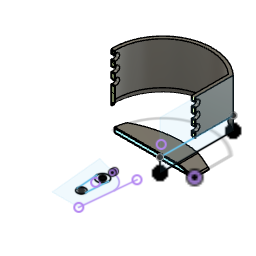
not a trashcan too v102 (Autodesk Fusion 360 design; units mm, degrees)
Autodesk Fusion 360 part; units mm, degrees
sketch "Sketch1" plane through (0, 0, 0) normal (0, 1, 0) x (1, 0, 0)
  circle A0 centre (0, 0) radius 35
  circle A1 centre (0, 0) radius 37.5
  line L0 (23, -29.6184) -> (23, 29.6184)
  line L1 (25.5, 27.4955) -> (25.5, -27.4955)
  dimension "d1" = 70
  dimension "d2" = 75
  dimension "d148" = 2.5
  dimension "d149" = 23
  constraint coincident A0.centre A1.centre
  constraint coincident A1 L0.start
  constraint coincident A1 L0.end
  constraint vertical L0
  constraint coincident A1 L1.start
  constraint coincident A1 L1.end
  constraint parallel L0 L1
  measures "d1" diameter of A0
  measures "d2" diameter of A1
  measures "d148" distance of L0 L1
  measures "d149" distance of A0.centre L0
extrude "Extrude1" add sketch "Sketch1" along normal blind 50 contours A0 L0 L1 | A0 A1 L0 L1 | A0 A1 L0 L1 | A0 A1 L0 makes body 1
ref_plane "WorkPlane2" through (0, 14, 0) normal (0, 1, 0) x (0, 0, 1)
sketch "Sketch4" plane through (0, 14, 0) normal (0, 1, 0) x (1, 0, 0)
  circle A0 centre (0, -68.5) radius 1.15
  circle A1 centre (0, -40.5) radius 1.15
  line L0 (-10, -36.1421) -> (10, -36.1421)
  line L1 (-10, -36.1421) -> (-10, -76.1421)
  line L2 (-10, -76.1421) -> (10, -76.1421)
  line L3 (10, -76.1421) -> (10, -36.1421)
  line L4 (-6.5, -43) -> (6.5, -43)
  line L5 (6.5, -43) -> (6.5, -66)
  line L6 (6.5, -66) -> (-6.5, -66)
  line L7 (-6.5, -66) -> (-6.5, -43)
  arc A2 (25.5, 27.4955) -> (25.5, -27.4955) centre (0, 0) ccw
  arc A3 (23, 26.3818) -> (23, -26.3818) centre (0, 0) ccw
  dimension "d28" = 2.3
  dimension "d29" = 2.3
  dimension "d30" = 28
  dimension "d33" = 40.5
  dimension "d36" = 20
  dimension "d37" = 40
  dimension "d38" = 10
  dimension "d39" = 10
  dimension "d40" = 13
  dimension "d41" = 23
  dimension "d42" = 3.5
  dimension "d43" = 2.5
  constraint coincident L0.start A2
  constraint coincident L0.end A2
  constraint horizontal L0
  constraint perpendicular L0 L1
  constraint perpendicular L1 L2
  constraint perpendicular L0 L3
  constraint horizontal L4
  constraint vertical L5
  constraint perpendicular L5 L6
  constraint perpendicular L4 L7
  measures "d28" diameter of A0
  measures "d29" diameter of A1
  measures "d30" distance of A0.centre A1.centre
  measures "d33" vertical distance of A1.centre A2.centre
  measures "d36" distance of L0.start L0.end
  measures "d37" distance of L0.start L1.end
  measures "d38" horizontal distance of A1.centre L0.start
  measures "d39" horizontal distance of A0.centre L0.start
  measures "d40" distance of L4.start L4.end
  measures "d41" distance of L4.end L5.end
  measures "d42" distance of L1 L7
  measures "d43" distance of A1.centre L4
extrude "Extrude2" add sketch "Sketch4" along normal blind 4 contours L1 L2 L3 A2 bodies 1
other "Base Mesh Feature1"
copy_body "Body->Comp1" bodies 1 removing the originals makes body 2 in component "Component"
ref_plane "WorkPlane3" through (0, -0.1, 0) normal (0, 1, 0) x (0, 0, 1)
sketch "Sketch8" plane through (0, -0.1, 0) normal (0, 1, 0) x (1, 0, 0)
  circle A0 centre (0, 0) radius 35
  line L0 (-13.92, -32.1128) -> (-10, -71.9203)
  line L1 (-10, -71.9203) -> (10, -71.9203)
  line L2 (10, -71.9203) -> (13.92, -32.1128)
  line L3 (0, 0) -> (24.0416, 24.0416)
  line L4 (0, 0) -> (34, 0) construction
  line L5 (0, 49.4975) -> (91.9239, -42.4264) construction
  line L6 (0, 49.4975) -> (-91.9239, -42.4264)
  line L7 (0, 0) -> (-24.0416, 24.0416)
  line L8 (0, 0) -> (34, 0) construction
  line L9 (0, -49.268) -> (67, -49.268) construction
  line L10 (0, -49.268) -> (70, -49.268) construction
  circle A1 centre (0, -49.268) radius 69.5542
  circle A2 centre (0, -49.268) radius 12.5
  line L11 (-0.0071, -36.768) -> (-0.0071, -35)
  point P0 (0, -49.268)
  dimension "d68" = 70
  dimension "d70" = 40
  dimension "d71" = 40
  dimension "d72" = 20
  dimension "d73" = 17
  dimension "d74" = 17
  dimension "d119" = 45
  dimension "d120" = 34
  dimension "d121" = 135
  dimension "d122" = 35
  dimension "d123" = 35
  dimension "d124" = 130
  dimension "d125" = 130
  dimension "d126" = 49.268
  dimension "d133" = 25
  constraint coincident A0.centre L3.start
  constraint coincident A0 L0.start
  constraint horizontal L1
  constraint coincident A0 L2.end
  constraint horizontal L4
  constraint perpendicular L3 L5
  constraint horizontal L8
  constraint perpendicular L6 L7
  constraint horizontal L9
  constraint coincident P0 L9.start
  constraint horizontal L10
  constraint concentric A1 A2
  constraint coincident A2 L11.start
  constraint coincident A0 L11.end
  constraint vertical L11
  measures "d68" diameter of A0
  measures "d70" distance of L0.start L0.end
  measures "d71" distance of L1.end L2.end
  measures "d72" distance of L0.end L1.end
  measures "d73" distance of A0.centre L0
  measures "d74" distance of A0.centre L2
  measures "d119" angle of L3 L4
  measures "d120" distance of A0.centre L3.end
  measures "d121" angle of L7 L8
  measures "d122" distance of A0.centre L6
  measures "d123" distance of A0.centre L5
  measures "d124" distance of L5.start L6.end
  measures "d125" distance of L5.start L5.end
  measures "d126" distance of A0.centre P0
  measures "d133" diameter of A2
extrude "Extrude5" add sketch "Sketch8" against normal blind 1 separate body contours A0 L3 L7 A1 | A0 L0 A2 L11 | A0 L2 A2 L11 | L0 L2 A2 | L3 L7 A1 | L0 L1 L2 A2 makes body 3
copy_body "Body->Comp2" bodies 3 removing the originals makes body 4 in component "Component'"
extrude "Extrude1'" add sketch "Sketch8" along normal blind 9 contours A0 L0 A2 L11 | L0 L2 A2 | L0 L1 L2 A2 bodies 4 in component "Component'"
sketch "Sketch9" plane through (0, 8.9, 0) normal (0, 1, 0) x (-1, 0, 0)
  line L0 (13.92, 32.1128) -> (10, 71.9203)
  line L1 (10, 71.9203) -> (-10, 71.9203)
  line L2 (-10, 71.9203) -> (-12.3921, 47.6289)
  arc A0 (13.92, 32.1128) -> (0.0071, 35) centre (0, 0) ccw
  circle A1 centre (0, 44) radius 4.25
  circle A2 centre (0, 60) radius 3
  line L3 (-10, 71.9203) -> (-13.92, 32.1128)
  line L4 (-2.9992, 59.9302) -> (-4.2494, 43.9302)
  line L5 (2.9992, 60.0698) -> (4.2494, 44.0698)
  circle A3 centre (0, 44) radius 1.75
  arc A4 (-12.3921, 47.6289) -> (0.0071, 36.768) centre (0, 49.268) ccw
  line L6 (0.0071, 36.768) -> (0.0071, 35)
  dimension "d81" = 8.5
  dimension "d84" = 44
  dimension "d86" = 6
  dimension "d87" = 16
  dimension "d93" = 16
  dimension "d94" = 16
  dimension "d95" = 8.936
  dimension "d96" = 3.5
  dimension "d135" = 10
  constraint coincident A2 L4.start
  constraint coincident A1 L4.end
  constraint coincident A2 L5.start
  constraint coincident A1 L5.end
  constraint equal L4 L5
  constraint concentric A1 A3
  measures "d81" diameter of A1
  measures "d84" vertical distance of A1.centre A0.centre
  measures "d86" diameter of A2
  measures "d87" vertical distance of A1.centre A2.centre
  measures "d93" vertical distance of L4.start L4.end
  measures "d94" vertical distance of L5.start L5.end
  measures "d95" angle of L4 L5
  measures "d96" diameter of A3
  measures "d135" horizontal distance of L0.end A1.centre
extrude "Extrude2'" cut sketch "Sketch9" against normal up to surface (10 mm away) contours A3 bodies 4 in component "Component'"
extrude "Extrude3" cut sketch "Sketch9" against normal blind 4.5 contours A1 L4 L5 | A1 A2 L4 L5 | A2 bodies 4 in component "Component'"
fillet "Fillet1" radius 6.5 2 edges at (-10, 3.9, 71.9203) (10, 3.9, 71.9203) on bodies 4 in component "Component'"
fillet "Fillet1'" radius 6.5 2 edges at (-10, 16, 76.1421) (10, 16, 76.1421) on bodies 2 in component "Component"
sketch "Sketch10" plane through (0, 0, 0) normal (1, 0, 0) x (0, 0, -1)
  circle A0 centre (0, 13) radius 2.5
  circle A1 centre (0, 45) radius 2.5
  circle A2 centre (0, 21) radius 2.5
  circle A3 centre (0, 29) radius 2.5
  circle A4 centre (0, 37) radius 2.5
  circle A5 centre (0, 5) radius 2.5
  dimension "d107" = 5
  dimension "d108" = 5
  dimension "d109" = 5
  dimension "d110" = 5
  dimension "d111" = 5
  dimension "d112" = 8
  dimension "d113" = 8
  dimension "d114" = 8
  dimension "d115" = 8
  dimension "d117" = 5
  dimension "d118" = 8
  measures "d107" diameter of A0
  measures "d108" diameter of A1
  measures "d109" diameter of A2
  measures "d110" diameter of A3
  measures "d111" diameter of A4
  measures "d112" distance of A0.centre A2.centre
  measures "d113" distance of A2.centre A3.centre
  measures "d114" distance of A3.centre A4.centre
  measures "d115" vertical distance of A1.centre A4.centre
  measures "d117" diameter of A5
  measures "d118" distance of A0.centre A5.centre
extrude "Extrude4" cut sketch "Sketch10" along normal through all and the other way through all contours A1 | A3 | A4 sketch seen with x (1, 0, 0) y (0, 1, 0) z (0, 0, 1) at (-0.1682, 0.5173, -0.0553) bodies 2 in component "Component"
copy_body "Body->Comp1'" bodies 2 removing the originals makes body 5 in component "Component''"
sketch "Sketch11" plane through (0, -1.1, 0) normal (0, -1, 0) x (1, 0, 0)
  arc A0 (10.5773, 66.0573) -> (4.1086, 71.9203) centre (4.1086, 65.4203) ccw
  line L0 (4.1086, 71.9203) -> (-4.1086, 71.9203)
  arc A1 (-4.1086, 71.9203) -> (-10.5773, 66.0573) centre (-4.1086, 65.4203) ccw
  line L1 (-10.5773, 66.0573) -> (-13.92, 32.1128)
  arc A2 (-13.92, 32.1128) -> (-32.8673, -12.0307) centre (0, 0) ccw
  arc A3 (-32.8673, -12.0307) -> (32.8673, -12.0307) centre (0, 49.268) ccw
  arc A4 (32.8673, -12.0307) -> (13.92, 32.1128) centre (0, 0) ccw
  line L2 (13.92, 32.1128) -> (10.5773, 66.0573)
  circle A5 centre (0, 44) radius 1.75
  circle A6 centre (0, 44) radius 2.75
  dimension "d130" = 5.5
  constraint concentric A5 A6
  measures "d130" diameter of A6
extrude "Extrude4'" cut sketch "Sketch11" against normal blind 2.5 contours A6 bodies 4 in component "Component'"
fillet "Fillet2" radius 39 2 edges at (-0.0071, 4.4, 35) (-0.0071, 4.4, 36.768) on bodies 4 in component "Component'"
extrude "Extrude5'" add 1 faces at (1.6288, -1.1, 14.7038) along direction (0, -1, 0) blind 2 on bodies 4 bodies 4 in component "Component'"
sketch "Sketch12" plane through (0, 0, 0) normal (1, 0, 0) x (0, 0, -1)
  line L0 (-39.2185, -5.1672) -> (-39.2185, 15.8328)
  line L1 (-39.2185, 15.8328) -> (41.5808, 15.8328)
  line L2 (41.5808, 15.8328) -> (41.5808, -5.1672)
  line L3 (41.5808, -5.1672) -> (-39.2185, -5.1672)
  dimension "d141" = 21
  constraint vertical L0
  constraint perpendicular L0 L1
  constraint perpendicular L1 L2
  constraint perpendicular L0 L3
  measures "d141" distance of L1.end L2.end
extrude "Extrude1''" cut sketch "Sketch12" along normal through all and the other way through all sketch seen with x (1, 0, 0) y (0, 1, 0) z (0, 0, 1) at (0.3396, -2.0002, 1.4447) bodies 5 in component "Component''"
extrude "Extrude6" add 1 faces at (2.3999, 1.4, 43.7764) along direction (0, -1, 0) blind 1.5 on bodies 4 bodies 4 in component "Component'"
other "Body->Comp1''"
fillet "Fillet1''" radius 58.5 2 edges at (10, 16, 36.1421) (-10, 16, 36.1421) on bodies 5 in component "Component''"
fillet "Fillet3" radius 4 4 edges at (-9.7907, -0.1, 33.6027) (-0.1713, -0.1, 35.8039) (5.0809, -0.1, 37.8458) (10.059, -0.1, 41.8474) on bodies 4 in component "Component'"
ref_plane "WorkPlane4" through (25, 0, 0) normal (1, 0, 0) x (0, 1, 0)
sketch "Sketch15" plane through (25, 0, 0) normal (1, 0, 0) x (0, 0, -1)
  line L0 (-38.3172, 6.5751) -> (18.4249, 6.5751)
  line L1 (18.4249, 6.5751) -> (18.4249, -5.2507)
  line L2 (18.4249, -5.2507) -> (-38.3172, -5.2507)
  line L3 (-38.3172, -5.2507) -> (-38.3172, 6.5751)
  constraint horizontal L0
  constraint vertical L1
  constraint horizontal L2
  constraint vertical L3
extrude "Extrude7" cut sketch "Sketch15" along normal blind 30 sketch seen with x (1, 0, 0) y (0, 1, 0) z (0, 0, 1) at (0.589, -2.5473, -4.2627) bodies 4 in component "Component'"
fillet "Fillet2'" radius 5 2 edges at (23, 13.8326, 0) (-35, 13.8326, 0) on bodies 5 in component "Component''"
chamfer "Chamfer1" distance 3 angle 45 1 edges at (25.589, -0.1, 4.2354) on bodies 4 in component "Component'"
chamfer "Chamfer2" distance 4 angle 45 1 edges at (22.589, -0.1, 5.1093) on bodies 4 in component "Component'"
chamfer "Chamfer3" distance 5 angle 45 1 edges at (18.589, -0.1, 5.9497) on bodies 4 in component "Component'"
chamfer "Chamfer4" distance 2.39 angle 45 1 edges at (23.2084, -2.0134, 4.9493) on bodies 4 in component "Component'"
chamfer "Chamfer5" distance 4.756 angle 45 1 edges at (20.8643, -1.5472, 5.5091) on bodies 4 in component "Component'"
chamfer "Chamfer6" distance 2.66 angle 45 1 edges at (16.1997, -0.6193, 6.3259) on bodies 4 in component "Component'"
chamfer "Chamfer7" distance 5.318 angle 45 1 edges at (18.78, -1.2656, 5.916) on bodies 4 in component "Component'"
sketch "Sketch18" plane through (25.1604, 0, 0) normal (1, 0, 0) x (0, 0, -1)
  line L0 (-26.0507, 15.8328) -> (28.9402, 15.8328)
  line L1 (28.9402, 15.8328) -> (28.9402, 52.0002)
  line L2 (28.9402, 52.0002) -> (-26.0507, 52.0002)
  line L3 (-26.0507, 52.0002) -> (-26.0507, 20.0002)
  line L4 (-26.0507, 20.0002) -> (-26.0507, 16.0002)
  line L5 (-26.0507, 16.0002) -> (-26.0507, 15.8328)
  circle A0 centre (1.5, 31.5174) radius 2.5
  circle A1 centre (1.5, 39.5174) radius 2.5
  circle A2 centre (1.5, 47.5174) radius 2.5
  line L6 (-26.0507, 15.8328) -> (-26.0507, 26.1563)
  line L7 (-26.0507, 26.1563) -> (28.9402, 25.8273)
  line L8 (28.9402, 15.8328) -> (-26.0507, 15.8328)
  dimension "d174" = 26
  constraint coincident L3 L6.end
  constraint coincident L0.start L5.end
  constraint coincident L1 L7.end
  constraint coincident L0.end L1.start
  measures "d174" distance of origin L7
extrude "Extrude3'" cut sketch "Sketch18" against normal blind 15 contours L0 L1 L3 L4 L5 L6 L7 L8 sketch seen with x (1, 0, 0) y (0, 1, 0) z (0, 0, 1) at (0.3396, -2.0002, 1.4447) bodies 5 in component "Component''"
chamfer "Chamfer2'" distance 1 angle 45 1 edges at (23, 23.9916, 0) on bodies 5 in component "Component''"
ref_plane "WorkPlane5" through (7, 0, 0) normal (1, 0, 0) x (0, 1, 0)
sketch "Sketch20" plane through (7, 0, 0) normal (1, 0, 0) x (0, 0, -1)
  line L0 (-26.0507, 20.0002) -> (-65.7149, 20.0002)
  line L1 (-24.8282, 20.0002) -> (-36.0553, 20.0002)
  line L2 (-26.0507, 20.0002) -> (-26.0507, 26.1563)
  line L3 (-26.0507, 26.1563) -> (-26.0507, 52.0002)
  line L4 (38.9447, 52.0002) -> (-36.0553, 52.0002)
  line L5 (28.9402, 52.0002) -> (28.9402, 25.8273)
  line L6 (28.9402, 25.8273) -> (28.9402, 15.8328)
  line L7 (38.9447, 15.8328) -> (-36.0553, 15.8328)
  line L8 (-26.0507, 15.8328) -> (-26.0507, 16.0002)
  line L9 (-36.0553, 16.0002) -> (-24.8282, 16.0002)
  line L10 (-24.8282, 16.0002) -> (-24.8282, 20.0002)
  spline S0 degree 3 poles (-1, 47.5174) (-1, 47.2034) (-0.9372, 46.8685) (-0.682, 46.2526) (-0.4897, 45.9716) (-0.0458, 45.5277) (0.2352, 45.3354) (0.8512, 45.0802) (1.186, 45.0174) (1.814, 45.0174) (2.1489, 45.0802) (2.7648, 45.3354) (3.0459, 45.5278) (3.4897, 45.9716) (3.6821, 46.2526) (3.9372, 46.8685) (4, 47.2034) (4, 47.5174) (4, 47.8314) (3.9372, 48.1663) (3.6821, 48.7822) (3.4897, 49.0633) (3.0459, 49.5071) (2.7648, 49.6995) (2.1489, 49.9547) (1.814, 50.0174) (1.186, 50.0174) (0.8511, 49.9547) (0.2352, 49.6995) (-0.0458, 49.5071) (-0.4897, 49.0633) (-0.6821, 48.7822) (-0.9372, 48.1663) (-1, 47.8314) (-1, 47.5174) knots 0.753614 0.753614 0.753614 0.753614 0.847815 0.847815 0.942016 0.942016 1.036214 1.036214 1.130412 1.130412 1.224618 1.224618 1.318823 1.318823 1.413025 1.413025 1.507227 1.507227 1.507227 1.60143 1.60143 1.695634 1.695634 1.789838 1.789838 1.884042 1.884042 1.978241 1.978241 2.072441 2.072441 2.166641 2.166641 2.260841 2.260841 2.260841 2.260841
  spline S1 degree 3 poles (-1, 39.5174) (-1, 39.2034) (-0.9372, 38.8685) (-0.682, 38.2526) (-0.4897, 37.9716) (-0.0458, 37.5277) (0.2352, 37.3354) (0.8512, 37.0802) (1.186, 37.0174) (1.814, 37.0174) (2.1489, 37.0802) (2.7648, 37.3354) (3.0459, 37.5278) (3.4897, 37.9716) (3.6821, 38.2526) (3.9372, 38.8685) (4, 39.2034) (4, 39.5174) (4, 39.8314) (3.9372, 40.1663) (3.6821, 40.7822) (3.4897, 41.0633) (3.0459, 41.5071) (2.7648, 41.6995) (2.1489, 41.9547) (1.814, 42.0174) (1.186, 42.0174) (0.8511, 41.9547) (0.2352, 41.6995) (-0.0458, 41.5071) (-0.4897, 41.0633) (-0.6821, 40.7822) (-0.9372, 40.1663) (-1, 39.8314) (-1, 39.5174) knots 0.753614 0.753614 0.753614 0.753614 0.847815 0.847815 0.942016 0.942016 1.036214 1.036214 1.130412 1.130412 1.224618 1.224618 1.318823 1.318823 1.413025 1.413025 1.507227 1.507227 1.507227 1.60143 1.60143 1.695634 1.695634 1.789838 1.789838 1.884042 1.884042 1.978241 1.978241 2.072441 2.072441 2.166641 2.166641 2.260841 2.260841 2.260841 2.260841
  spline S2 degree 3 poles (-1, 31.5174) (-1, 31.2034) (-0.9372, 30.8685) (-0.682, 30.2526) (-0.4897, 29.9716) (-0.0458, 29.5277) (0.2352, 29.3354) (0.8512, 29.0802) (1.186, 29.0174) (1.814, 29.0174) (2.1489, 29.0802) (2.7648, 29.3354) (3.0459, 29.5278) (3.4897, 29.9716) (3.6821, 30.2526) (3.9372, 30.8685) (4, 31.2034) (4, 31.5174) (4, 31.8314) (3.9372, 32.1663) (3.6821, 32.7822) (3.4897, 33.0633) (3.0459, 33.5071) (2.7648, 33.6995) (2.1489, 33.9547) (1.814, 34.0174) (1.186, 34.0174) (0.8511, 33.9547) (0.2352, 33.6995) (-0.0458, 33.5071) (-0.4897, 33.0633) (-0.6821, 32.7822) (-0.9372, 32.1663) (-1, 31.8314) (-1, 31.5174) knots 0.753614 0.753614 0.753614 0.753614 0.847815 0.847815 0.942016 0.942016 1.036214 1.036214 1.130412 1.130412 1.224618 1.224618 1.318823 1.318823 1.413025 1.413025 1.507227 1.507227 1.507227 1.60143 1.60143 1.695634 1.695634 1.789838 1.789838 1.884042 1.884042 1.978241 1.978241 2.072441 2.072441 2.166641 2.166641 2.260841 2.260841 2.260841 2.260841
  line L11 (-65.7149, 20.0002) -> (-34.4899, 45.0002)
  line L12 (-34.4899, 45.0002) -> (-34.6309, 20.0002)
  dimension "d178" = 25
  dimension "d179" = 40
  constraint coincident L0.end L11.start
  constraint coincident L1 L12.end
  measures "d178" vertical distance of L11.end L12.end
  measures "d179" distance of L0.end L11.end
extrude "Extrude4''" add sketch "Sketch20" along normal blind 2 contours L0 L1 L11 L12 sketch seen with x (1, 0, 0) y (0, 1, 0) z (0, 0, 1) at (0.3396, -2.0002, 1.4447) bodies 5 in component "Component''"
ref_plane "WorkPlane6" through (-7, 0, 0) normal (1, 0, 0) x (0, 1, 0)
sketch "Sketch21" plane through (-7, 0, 0) normal (1, 0, 0) x (0, 0, -1)
  line L0 (-24.8282, 20.0002) -> (-65.8141, 20.0002)
  line L1 (-65.8141, 20.0002) -> (-34.5891, 45.0002)
  line L2 (-34.5891, 20.0002) -> (-34.5891, 45.0002)
  dimension "d181" = 40
  dimension "d182" = 25
  constraint coincident L0.end L1.start
  constraint coincident L0 L2.start
  constraint perpendicular L0 L2
  measures "d181" distance of L0.end L1.end
  measures "d182" distance of L1.end L2.start
extrude "Extrude5''" add sketch "Sketch21" against normal blind 2 sketch seen with x (1, 0, 0) y (0, 1, 0) z (0, 0, 1) at (0.3396, -2.0002, 1.4447) bodies 5 in component "Component''"
chamfer "Chamfer3'" distance 10 angle 45 2 edges at (9.3396, 30.3464, 36.3183) (-8.6604, 30.3189, 36.4863) on bodies 5 in component "Component''"
component "Component" placed x (1, 0, 0) y (0, 1, 0) z (0, 0, 1) at (0.1682, -0.5173, 0.0553)
component "Component'" placed x (1, 0, 0) y (0, 1, 0) z (0, 0, 1) at (-0.589, 2.5473, 4.2627)
component "servo_MG90S" placed x (1, 0, 0) y (0, 1, 0) z (0, 0, 1) at (-0.442, 6.1032, 1.3879)
component "Component''" placed x (1, 0, 0) y (0, 1, 0) z (0, 0, 1) at (-0.5078, 2.5174, -1.5) in component "Component"
